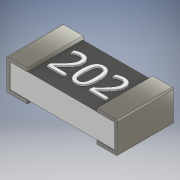
# Autodesk Inventor part: 21-1001
Saved by Autodesk Inventor 2018 (Build 220112000, 112)
## iProperties
Created: 2019-09-21
Part Number: 21-1001
Material: Copper
Document SubType Name: Modeling
Designer: Bradley
Density: 8.94 g/cm^3
Appearance: Smooth - White
Author: Bradley
Autodesk Inventor part; units mm, degrees
ref_plane "YZ Plane" through (0, 0, 0) normal (1, 0, 0) x (0, 1, 0)
ref_plane "XZ Plane" through (0, 0, 0) normal (0, 1, 0) x (-1, 0, 0)
ref_plane "XY Plane" through (0, 0, 0) normal (0, 0, 1) x (1, 0, 0)
sketch "Sketch1" plane through (0, 0, 0) normal (0, 1, 0) x (-1, 0, 0)
  line L0 (0.75, 0.175) -> (-0.75, 0.175)
  line L1 (-0.75, 0.175) -> (-0.75, -0.175)
  line L2 (-0.75, -0.175) -> (0.75, -0.175)
  line L3 (0.75, -0.175) -> (0.75, 0.175)
  line L4 (0.5, 0.175) -> (0.5, 0.225)
  line L5 (0.5, 0.225) -> (0.8, 0.225)
  line L6 (0.8, 0.225) -> (0.8, -0.225)
  line L7 (0.8, -0.225) -> (0.5, -0.225)
  line L8 (0.5, -0.225) -> (0.5, -0.175)
  line L9 (-0.5, 0.175) -> (-0.5, 0.225)
  line L10 (-0.5, 0.225) -> (-0.8, 0.225)
  line L11 (-0.8, 0.225) -> (-0.8, -0.225)
  line L12 (-0.8, -0.225) -> (-0.5, -0.225)
  line L13 (-0.5, -0.175) -> (-0.5, -0.225)
  line L14 (0.5, 0.175) -> (-0.5, 0.175)
  point P0 (0, 0)
  point P1 (0, 0.175)
  point P2 (0.75, 0)
  dimension "d0" = 1.6
  dimension "d1" = 0.05
  dimension "d2" = 0.05
  dimension "d3" = 0.45
  dimension "d4" = 0.3
  constraints: 30 end point, 12 point on line, 7 perpendicular, 3 collinear, 3 midpoint, 2 parallel, 1 horizontal, 1 horizontal alignment, 1 vertical, 1 vertical alignment
  measures "d0" distance between parallel lines of L11 L6
  measures "d1" distance of L7.end L8.end
  measures "d2" distance between parallel lines of L6 L3
  measures "d3" distance of L5.end L6.end
  measures "d4" distance of L6.end L7.end
extrude "Extrusion1" add sketch "Sketch1" along normal mid plane 0.8 contours L0 L4 L5 L6 L7 L8 L2 L3 | L0 L1 L2 L13 L12 L11 L10 L9
extrude "Extrusion2" add sketch "Sketch1" along normal mid plane 0.79 contours L3 L2 L1 L0
sketch "Sketch2" plane through (-0.5, -0.395, 0.175) normal (0, 0, 1) x (1, 0, 0)
  line L0 (0, 0) -> (0, 0.79) projected
  line L1 (1, 0) -> (0, 0) projected
  line L2 (1, 0) -> (1, 0.79) projected
  line L3 (0, 0.79) -> (1, 0.79) projected
  line L4 (0, 0.395) -> (1, 0.395) construction
  line L5 (0.3256, 0.195) -> (0.0789, 0.195)
  line L6 (0.0789, 0.195) -> (0.0789, 0.2517)
  spline S0 degree 2 poles (0.0789, 0.2517) (0.1055, 0.2767) (0.1528, 0.323) (0.1755, 0.348) knots 0 0 0 1 2 2 2
  spline S1 degree 2 poles (0.1755, 0.348) (0.2212, 0.3982) (0.2546, 0.4585) (0.2546, 0.4906) knots 0 0 0 1 2 2 2
  spline S2 degree 2 poles (0.2546, 0.4906) (0.2546, 0.5075) (0.2442, 0.5328) (0.2348, 0.5409) knots 0 0 0 1 2 2 2
  spline S3 degree 2 poles (0.2348, 0.5409) (0.2254, 0.549) (0.2008, 0.5571) (0.1859, 0.5571) knots 0 0 0 1 2 2 2
  spline S4 degree 2 poles (0.1859, 0.5571) (0.1716, 0.5571) (0.1425, 0.5499) (0.1292, 0.5444) knots 0 0 0 1 2 2 2
  spline S5 degree 2 poles (0.1292, 0.5444) (0.1178, 0.5399) (0.0968, 0.5269) (0.0903, 0.5224) knots 0 0 0 1 2 2 2
  line L7 (0.0903, 0.5224) -> (0.0874, 0.5224)
  line L8 (0.0874, 0.5224) -> (0.0874, 0.5794)
  spline S6 degree 2 poles (0.0874, 0.5794) (0.1039, 0.5875) (0.1632, 0.6034) (0.1898, 0.6034) knots 0 0 0 1 2 2 2
  spline S7 degree 2 poles (0.1898, 0.6034) (0.2459, 0.6034) (0.3091, 0.5441) (0.3091, 0.4935) knots 0 0 0 1 2 2 2
  spline S8 degree 2 poles (0.3091, 0.4935) (0.3091, 0.4699) (0.2981, 0.4303) (0.2883, 0.4135) knots 0 0 0 1 2 2 2
  spline S9 degree 2 poles (0.2883, 0.4135) (0.2786, 0.396) (0.2504, 0.3616) (0.2348, 0.3451) knots 0 0 0 1 2 2 2
  spline S10 degree 2 poles (0.2348, 0.3451) (0.2096, 0.3175) (0.1476, 0.2585) (0.1292, 0.2414) knots 0 0 0 1 2 2 2
  line L9 (0.1292, 0.2414) -> (0.3256, 0.2414)
  line L10 (0.3256, 0.2414) -> (0.3256, 0.195)
  spline S11 degree 2 poles (0.628, 0.395) (0.628, 0.2874) (0.5655, 0.1866) (0.5003, 0.1866) knots 0 0 0 1 2 2 2
  spline S12 degree 2 poles (0.5003, 0.1866) (0.4342, 0.1866) (0.3723, 0.2893) (0.3723, 0.3947) knots 0 0 0 1 2 2 2
  spline S13 degree 2 poles (0.3723, 0.3947) (0.3723, 0.5029) (0.4348, 0.6031) (0.5003, 0.6031) knots 0 0 0 1 2 2 2
  spline S14 degree 2 poles (0.5003, 0.6031) (0.5661, 0.6031) (0.628, 0.4994) (0.628, 0.395) knots 0 0 0 1 2 2 2
  spline S15 degree 2 poles (0.5593, 0.2731) (0.5671, 0.2929) (0.5736, 0.3538) (0.5736, 0.395) knots 0 0 0 1 2 2 2
  spline S16 degree 2 poles (0.5736, 0.395) (0.5736, 0.4362) (0.5671, 0.4968) (0.559, 0.5172) knots 0 0 0 1 2 2 2
  spline S17 degree 2 poles (0.559, 0.5172) (0.5509, 0.5376) (0.5227, 0.5587) (0.5003, 0.5587) knots 0 0 0 1 2 2 2
  spline S18 degree 2 poles (0.5003, 0.5587) (0.478, 0.5587) (0.4491, 0.5376) (0.4407, 0.5166) knots 0 0 0 1 2 2 2
  spline S19 degree 2 poles (0.4407, 0.5166) (0.4326, 0.4961) (0.4267, 0.4339) (0.4267, 0.3947) knots 0 0 0 1 2 2 2
  spline S20 degree 2 poles (0.4267, 0.3947) (0.4267, 0.3525) (0.4319, 0.2961) (0.4404, 0.2741) knots 0 0 0 1 2 2 2
  spline S21 degree 2 poles (0.4404, 0.2741) (0.4481, 0.2533) (0.477, 0.231) (0.5003, 0.231) knots 0 0 0 1 2 2 2
  spline S22 degree 2 poles (0.5003, 0.231) (0.5224, 0.231) (0.5512, 0.2521) (0.5593, 0.2731) knots 0 0 0 1 2 2 2
  line L11 (0.9259, 0.195) -> (0.6793, 0.195)
  line L12 (0.6793, 0.195) -> (0.6793, 0.2517)
  spline S23 degree 2 poles (0.6793, 0.2517) (0.7058, 0.2767) (0.7532, 0.323) (0.7759, 0.348) knots 0 0 0 1 2 2 2
  spline S24 degree 2 poles (0.7759, 0.348) (0.8216, 0.3982) (0.8549, 0.4585) (0.8549, 0.4906) knots 0 0 0 1 2 2 2
  spline S25 degree 2 poles (0.8549, 0.4906) (0.8549, 0.5075) (0.8446, 0.5328) (0.8352, 0.5409) knots 0 0 0 1 2 2 2
  spline S26 degree 2 poles (0.8352, 0.5409) (0.8258, 0.549) (0.8011, 0.5571) (0.7862, 0.5571) knots 0 0 0 1 2 2 2
  spline S27 degree 2 poles (0.7862, 0.5571) (0.772, 0.5571) (0.7428, 0.5499) (0.7295, 0.5444) knots 0 0 0 1 2 2 2
  spline S28 degree 2 poles (0.7295, 0.5444) (0.7182, 0.5399) (0.6971, 0.5269) (0.6906, 0.5224) knots 0 0 0 1 2 2 2
  line L13 (0.6906, 0.5224) -> (0.6877, 0.5224)
  line L14 (0.6877, 0.5224) -> (0.6877, 0.5794)
  spline S29 degree 2 poles (0.6877, 0.5794) (0.7042, 0.5875) (0.7635, 0.6034) (0.7901, 0.6034) knots 0 0 0 1 2 2 2
  spline S30 degree 2 poles (0.7901, 0.6034) (0.8462, 0.6034) (0.9094, 0.5441) (0.9094, 0.4935) knots 0 0 0 1 2 2 2
  spline S31 degree 2 poles (0.9094, 0.4935) (0.9094, 0.4699) (0.8984, 0.4303) (0.8887, 0.4135) knots 0 0 0 1 2 2 2
  spline S32 degree 2 poles (0.8887, 0.4135) (0.8789, 0.396) (0.8507, 0.3616) (0.8352, 0.3451) knots 0 0 0 1 2 2 2
  spline S33 degree 2 poles (0.8352, 0.3451) (0.8099, 0.3175) (0.748, 0.2585) (0.7295, 0.2414) knots 0 0 0 1 2 2 2
  line L15 (0.7295, 0.2414) -> (0.9259, 0.2414)
  line L16 (0.9259, 0.2414) -> (0.9259, 0.195)
  point P0 (0.5, 0.395)
  constraints: 2 end point, 2 midpoint, 1 horizontal
extrude "Extrusion3" add sketch "Sketch2" along normal blind 0.02 contours L5 L6 S0 S1 S2 S3 S4 S5 L7 L8 S6 S7 S8 S9 S10 L9 L10 | S11 S12 S13 S14 | L11 L12 S23 S24 S25 S26 S27 S28 L13 L14 S29 S30 S31 S32 S33 L15 L16
fillet "Fillet1" radius 0.02 4 edges at (-0.8, 0, 0.225) (-0.8, 0, -0.225) (0.8, 0, 0.225) (0.8, 0, -0.225)
equation "\"d2\" = d1"
body "Solid1"
